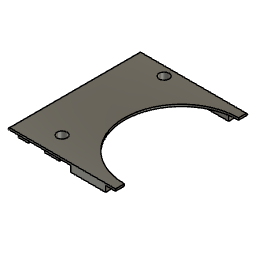
로봇팔 왼쪽 외장 (Autodesk Fusion 360 design; units mm, degrees)
Autodesk Fusion 360 part; units mm, degrees
note: some values were not read from the file. Set by a fixed rule: which sketch regions a step uses.
sketch "스케치1" plane through (0, 0, 0) normal (0, 0, 1) x (1, 0, 0)
  line L0 (0, 0) -> (-66.25, 0)
  line L1 (-66.25, 0) -> (-107.5, 0)
  circle A0 centre (0, 0) radius 57.35
  line L2 (0, 57.35) -> (0, -57.35)
  line L3 (0, 0) -> (0, 66.25)
  line L4 (0, 66.25) -> (-107.5, 66.25)
  line L5 (-107.5, 66.25) -> (-107.5, 46.25)
  line L6 (-107.5, 46.25) -> (-107.5, -36.25)
  line L7 (-107.5, -36.25) -> (-107.5, -56.25)
  line L8 (0, 0) -> (0, -66.25)
  line L9 (0, -66.25) -> (-107.5, -66.25)
  line L10 (-107.5, -56.25) -> (-107.5, -66.25)
  line L11 (-66.25, 66.25) -> (-66.25, -66.25)
  line L12 (-66.25, 66.25) -> (-81.25, 66.25)
  line L13 (-81.25, 66.25) -> (-81.25, 46.25)
  line L14 (-81.25, 46.25) -> (-66.25, 46.25)
  line L15 (-66.25, 46.25) -> (-66.25, 66.25)
  line L16 (-107.5, 66.25) -> (-97.5, 66.25)
  line L17 (-97.5, 66.25) -> (-97.5, 46.25)
  line L18 (-97.5, 46.25) -> (-107.5, 46.25)
  line L19 (-107.5, 46.25) -> (-107.5, 66.25)
  line L20 (-107.5, -36.25) -> (-66.25, -36.25)
  line L21 (-66.25, -36.25) -> (-66.25, -56.25)
  line L22 (-66.25, -56.25) -> (-107.5, -56.25)
  line L23 (-107.5, -56.25) -> (-107.5, -36.25)
  line L24 (-66.25, -36.25) -> (-81.25, -36.25)
  line L25 (-81.25, -36.25) -> (-81.25, -56.25)
  line L26 (-81.25, -56.25) -> (-66.25, -56.25)
  line L27 (-66.25, -56.25) -> (-66.25, -36.25)
  line L28 (-107.5, -36.25) -> (-97.5, -36.25)
  line L29 (-97.5, -36.25) -> (-97.5, -56.25)
  line L30 (-97.5, -56.25) -> (-107.5, -56.25)
  line L31 (-107.5, -56.25) -> (-107.5, -36.25)
  circle A1 centre (-73.75, 56.25) radius 2.6
  circle A2 centre (-73.75, -46.25) radius 2.6
  circle A3 centre (-73.75, 56.25) radius 5
  circle A4 centre (-73.75, -46.25) radius 5
  line L32 (-66.25, 66.25) -> (-56.25, 66.25)
  line L33 (-56.25, 66.25) -> (-56.25, 56.25)
  line L34 (-56.25, 56.25) -> (-66.25, 56.25)
  line L35 (-66.25, 56.25) -> (-66.25, 66.25)
  circle A5 centre (-56.25, 56.25) radius 5
  line L36 (-66.25, -66.25) -> (-56.25, -66.25)
  line L37 (-56.25, -66.25) -> (-56.25, -46.25)
  line L38 (-56.25, -46.25) -> (-66.25, -46.25)
  line L39 (-66.25, -46.25) -> (-66.25, -66.25)
  circle A6 centre (-56.25, -46.25) radius 5
  line L40 (0, -66.25) -> (-45, -66.25)
  line L41 (-45, -66.25) -> (-45, -57.35)
  line L42 (-45, -57.35) -> (0, -57.35)
  line L43 (0, -57.35) -> (0, -66.25)
  line L44 (0, -66.25) -> (-10, -66.25)
  line L45 (-10, -66.25) -> (-10, -57.35)
  line L46 (-10, -57.35) -> (0, -57.35)
  line L47 (0, -57.35) -> (0, -66.25)
  line L48 (0, 66.25) -> (-45, 66.25)
  line L49 (-45, 66.25) -> (-45, 57.35)
  line L50 (-45, 57.35) -> (0, 57.35)
  line L51 (0, 57.35) -> (0, 66.25)
  line L52 (0, 66.25) -> (-10, 66.25)
  line L53 (-10, 66.25) -> (-10, 57.35)
  line L54 (-10, 57.35) -> (0, 57.35)
  line L55 (0, 57.35) -> (0, 66.25)
  dimension "d1" = 66.25
  dimension "d2" = 41.25
  dimension "d3" = 114.7
  dimension "d4" = 66.25
  dimension "d5" = 20
  dimension "d6" = 82.5
  dimension "d7" = 20
  dimension "d8" = 66.25
  dimension "d9" = 15
  dimension "d10" = 20
  dimension "d11" = 10
  dimension "d12" = 20
  dimension "d13" = 20
  dimension "d14" = 15
  dimension "d15" = 20
  dimension "d16" = 10
  dimension "d17" = 5.2
  dimension "d18" = 5.2
  dimension "d19" = 10
  dimension "d20" = 10
  dimension "d21" = 10
  dimension "d22" = 10
  dimension "d23" = 10
  dimension "d24" = 10
  dimension "d25" = 20
  dimension "d26" = 10
  dimension "d31" = 45
  dimension "d32" = 10
  dimension "d35" = 45
  dimension "d36" = 10
  constraint coincident L0.start A0.centre
  constraint horizontal L0
  constraint parallel L0 L1
  constraint coincident A0 L2.start
  constraint coincident A0 L2.end
  constraint perpendicular L0 L2
  constraint perpendicular L0 L3
  constraint perpendicular L3 L4
  constraint perpendicular L4 L5
  constraint perpendicular L4 L6
  constraint vertical L7
  constraint perpendicular L0 L8
  constraint perpendicular L7 L9
  constraint perpendicular L9 L10
  constraint coincident L4 L11.start
  constraint coincident L9 L11.end
  constraint perpendicular L9 L11
  constraint horizontal L12
  constraint vertical L13
  constraint horizontal L14
  constraint vertical L15
  constraint horizontal L16
  constraint vertical L17
  constraint horizontal L18
  constraint vertical L19
  constraint horizontal L20
  constraint vertical L21
  constraint horizontal L22
  constraint vertical L23
  constraint horizontal L24
  constraint vertical L25
  constraint horizontal L26
  constraint vertical L27
  constraint horizontal L28
  constraint vertical L29
  constraint horizontal L30
  constraint vertical L31
  constraint concentric A1 A3
  constraint concentric A2 A4
  constraint horizontal L32
  constraint vertical L33
  constraint horizontal L34
  constraint vertical L35
  constraint coincident L33.end L34.start
  constraint horizontal L36
  constraint vertical L37
  constraint horizontal L38
  constraint vertical L39
  constraint coincident L37.end L38.start
  constraint horizontal L40
  constraint vertical L41
  constraint horizontal L42
  constraint vertical L43
  constraint horizontal L44
  constraint vertical L45
  constraint horizontal L46
  constraint vertical L47
  constraint coincident L42 L45.end
  constraint horizontal L48
  constraint vertical L49
  constraint horizontal L50
  constraint vertical L51
  constraint horizontal L52
  constraint vertical L53
  constraint horizontal L54
  constraint vertical L55
  measures "d1" distance of L0.start L0.end
  measures "d2" distance of L0.end L1.end
  measures "d3" diameter of A0
  measures "d4" distance of L0.start L3.end
  measures "d5" distance of L4.end L5.end
  measures "d6" distance of L5.end L6.end
  measures "d7" distance of L6.end L7.end
  measures "d8" distance of L0.start L8.end
  measures "d9" distance of L11.start L12.end
  measures "d10" distance of L11.start L14.end
  measures "d11" distance of L4.end L16.end
  measures "d12" distance of L4.end L5.end
  measures "d13" distance of L6.end L7.end
  measures "d14" distance of L20.end L24.end
  measures "d15" distance of L20.end L21.end
  measures "d16" distance of L6.end L28.end
  measures "d17" diameter of A1
  measures "d18" diameter of A2
  measures "d19" diameter of A3
  measures "d20" diameter of A4
  measures "d21" distance of L11.start L32.end
  measures "d22" distance of L11.start L34.end
  measures "d23" diameter of A5
  measures "d24" distance of L11.end L36.end
  measures "d25" distance of L11.end L38.end
  measures "d26" diameter of A6
  measures "d31" distance of L8.end L40.end
  measures "d32" distance of L8.end L44.end
  measures "d35" distance of L3.end L48.end
  measures "d36" distance of L3.end L52.end
extrude "돌출1" add sketch "스케치1" along normal blind 2 contours L0 A0 L9 L11 L21 L27 L37 L38 A6 L41 L42 L46 | L0 A0 L4 L11 L15 L33 L34 A5 L49 L50 L54 | L3 L4 L48 L50 L51 L52 L53 L54 L55 | L8 L9 L40 L42 L43 L44 L45 L46 L47 | L1 L6 L11 L20 L24 L28 | L1 L4 L6 L11 L13 L14 L17 L18 | L4 L48 L49 L50 L53 | L9 L40 L41 L42 L45 | L4 L11 L12 L13 L14 L15 L35 | L11 L20 L21 L22 L24 L25 L26 L27 L39 | L4 L5 L16 L17 L18 L19 | L7 L20 L22 L23 L28 L29 L30 L31 | L4 L11 L15 L32 L33 L34 L35 A5 | L9 L11 L21 L27 L36 L37 L38 L39 A6 | L20 L22 L25 L29 | L9 L10 L11 L22 L26 L30 L39 | L33 L34 A5 | L33 L34 A5 | L37 L38 A6 | L37 L38 A6
extrude "돌출2" add sketch "스케치1" against normal blind 12 contours L4 L11 L12 L13 L14 L15 L35 | L11 L20 L21 L22 L24 L25 L26 L27 L39 | L4 L5 L16 L17 L18 L19 | L7 L20 L22 L23 L28 L29 L30 L31 | A3 | A4
extrude "돌출3" add sketch "스케치1" against normal blind 6 contours L4 L48 L49 L50 L53 | L9 L40 L41 L42 L45
extrude "돌출4" cut 2 faces at (-69.5686, 56.0016, 0) (-69.5686, -46.4984, 0) along direction (0, 0, -1) blind 9
fillet "필렛2" radius 1 2 edges at (-53.75, 66.25, 2) (-107.5, 0, 2)
